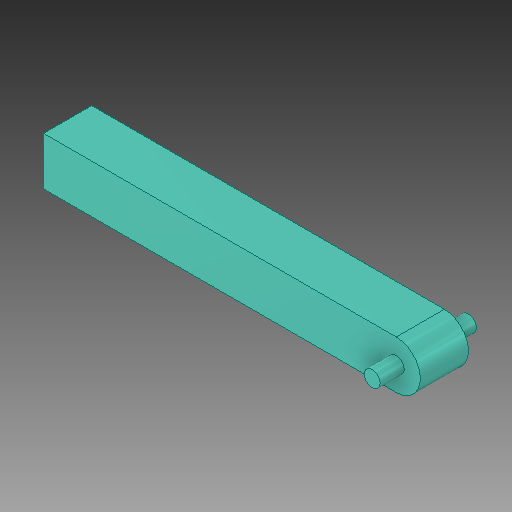
# Autodesk Inventor part: Arm
Saved by Autodesk Inventor 2018 (Build 220112000, 112)
## iProperties
Created: 2017-12-31
Part Number: Arm
Material: Generic
Document SubType Name: Modeling
Designer: suchanek
Density: 1 g/cm^3
Appearance: Default
Mass: 1.68767 g
Surface Area: 12.1452 cm^2
Volume: 1.68767 cm^3
Author: suchanek
Autodesk Inventor part; units mm, degrees
ref_plane "YZ Plane" through (0, 0, 0) normal (1, 0, 0) x (0, 1, 0)
ref_plane "XZ Plane" through (0, 0, 0) normal (0, 1, 0) x (-1, 0, 0)
ref_plane "XY Plane" through (0, 0, 0) normal (0, 0, 1) x (1, 0, 0)
sketch "Sketch1" plane through (0, 0, 0) normal (0, 0, 1) x (1, 0, 0)
  line L0 (0, 6) -> (47, 6)
  line L1 (56, 0) -> (0, 0)
  line L2 (47, 0) -> (47, 6)
  circle A0 centre (44, 3) radius 1
  line L3 (0, 0) -> (0, 6)
  arc A1 (44, 0) -> (44, 6) centre (44, 3) ccw
  dimension "d26" = 2
  dimension "d29" = 47
  dimension "d30" = 3
  dimension "d31" = 3
  dimension "d32" = 6
  constraints: 8 end point, 7 point on line, 2 centre point, 2 point on circle, 1 coincident, 1 horizontal, 1 parallel, 1 perpendicular, 1 vertical alignment
  measures "d26" diameter of A0
  measures "d29" distance between parallel lines of L3 L2
  measures "d30" distance from line of L2 A0.centre
  measures "d31" distance from line of L0 A0.centre
  measures "d32" distance between parallel lines of L0 L1
extrude "Extrusion1" add sketch "Sketch1" along normal mid plane 6 contours L0 A1 L1 L3 | A0
sketch "Sketch6" plane through (0, 0, 3) normal (0, 0, 1) x (1, 0, 0)
  line L0 (0, 6) -> (47, 6)
  line L1 (47, 0) -> (47, 6)
  circle A0 centre (44, 3) radius 1
  line L2 (0, 0) -> (0, 6)
  arc A1 (44, 0) -> (44, 6) centre (44, 3) ccw projected
  line L3 (0, 0) -> (44, 0) projected
  line L4 (44, 6) -> (0, 6) projected
  dimension "d34" = 2
  dimension "d36" = 3
  dimension "d37" = 3
  constraints: 6 end point, 4 point on line, 2 perpendicular, 1 centre point, 1 collinear, 1 horizontal, 1 tangent
  measures "d34" diameter of A0
  measures "d36" distance from line of L1 A0.centre
  measures "d37" distance from line of L0 A0.centre
extrude "Extrusion4" add sketch "Sketch6" along normal blind 3 and the other way blind 9 contours A0
body "Solid1"
